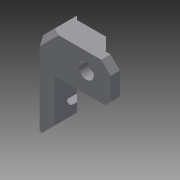
# Autodesk Inventor part: z-axis-top
Saved by Autodesk Inventor 2015 (Build 190159000, 159)
## iProperties
Created: 2015-05-31
Part Number: z-axis-top
Material: Generic
Document SubType Name: Modeling
Designer: X
Density: 1 g/cm^3
Appearance: Default
Author: X
Autodesk Inventor part; units mm, degrees
ref_plane "YZ Plane" through (0, 0, 0) normal (1, 0, 0) x (0, 1, 0)
ref_plane "XZ Plane" through (0, 0, 0) normal (0, 1, 0) x (-1, 0, 0)
ref_plane "XY Plane" through (0, 0, 0) normal (0, 0, 1) x (1, 0, 0)
sketch "Sketch1" plane through (0, 0, 0) normal (0, 1, 0) x (-1, 0, 0)
  line L0 (0, 0) -> (38, 0)
  line L1 (38, 0) -> (38, -50)
  line L2 (38, -50) -> (0, -50)
  line L3 (0, -50) -> (0, 0)
  dimension "d0" = 38
  dimension "d1" = 50
  constraints: 8 end point, 2 parallel, 1 horizontal, 1 perpendicular
  measures "d0" distance of L0.start L0.end
  measures "d1" distance of L2.end L0.start
extrude "Extrusion1" add sketch "Sketch1" along normal blind 16
sketch "Sketch2" plane through (0, 16, 0) normal (0, 1, 0) x (1, 0, 0)
  line L0 (0, 50) -> (-30, 50)
  line L1 (-30, 50) -> (-30, 20)
  line L2 (-30, 20) -> (0, 20)
  line L3 (0, 20) -> (0, 50)
  line L4 (-38, 50) -> (-38, 0) projected
  line L5 (0, 0) -> (-38, 0) projected
  dimension "d4" = 8
  dimension "d5" = 20
  constraints: 8 end point, 2 parallel, 1 horizontal, 1 perpendicular
  measures "d4" distance between parallel lines of L1 L4
  measures "d5" distance between parallel lines of L5 L2
extrude "Extrusion2" cut sketch "Sketch2" against normal through all
sketch "Sketch3" plane through (0, 16, 0) normal (0, 1, 0) x (1, 0, 0)
  line L0 (0, 20) -> (-30, 20)
  line L1 (-30, 20) -> (-30, 5)
  line L2 (-30, 5) -> (0, 5)
  line L3 (0, 5) -> (0, 20)
  line L4 (-30, 20) -> (-30, 50) projected
  line L5 (-38, 0) -> (0, 0) projected
  dimension "d8" = 5
  constraints: 8 end point, 2 parallel, 1 collinear, 1 horizontal, 1 perpendicular
  measures "d8" distance between parallel lines of L5 L2
extrude "Extrusion3" cut sketch "Sketch3" against normal blind 11
sketch "Sketch4" plane through (-38, 0, 0) normal (0, 0, 1) x (1, 0, 0)
  line L0 (4, 16) -> (8, 12)
  line L1 (8, 12) -> (23.5, 12)
  line L2 (23.5, 12) -> (30, 5.5)
  line L3 (30, 5.5) -> (30, 5)
  line L4 (30, 5) -> (38, 5)
  line L5 (4, 16) -> (38, 16)
  line L6 (38, 5) -> (38, 16) projected
  line L7 (38, 16) -> (38, 5)
  line L8 (0, 16) -> (38, 16) projected
  line L9 (38, 0) -> (38, 16) projected
  line L10 (38, 0) -> (0, 0) projected
  line L11 (0, 0) -> (0, 16) projected
  dimension "d11" = 0.5
  dimension "d12" = 8
  dimension "d13" = 5
  dimension "d16" = 7
  dimension "d17" = 15.5
  dimension "d18" = 8
  dimension "d19" = 4
  constraints: 14 end point, 2 perpendicular, 1 collinear, 1 horizontal, 1 parallel, 1 point on line, 1 vertical
  measures "d11" distance of L2.end L3.end
  measures "d12" distance of L3.end L4.end
  measures "d13" distance between parallel lines of L10 L4
  measures "d16" distance from line of L3.end L1
  measures "d17" distance of L0.end L1.end
  measures "d18" distance from line of L11 L0.end
  measures "d19" distance from line of L11 L0.start
extrude "Extrusion4" cut sketch "Sketch4" against normal through all contours L5 L6 L4 L3 L2 L1 L0
chamfer "Chamfer1" distance 7 distance2 7 1 edges at (-30, 6, -50) measured on face at (-30.5, 6, -50)
chamfer "Chamfer2" distance 6 distance2 6 1 edges at (-38, 8, 0) measured on face at (-38, 8, -0.5)
chamfer "Chamfer3" distance 1 distance2 1 1 edges at (-38, 8, -50) measured on face at (-37.5, 8, -50)
chamfer "Chamfer4" distance 5 distance2 5 1 edges at (0, 2.5, 0) measured on face at (-0.5, 2.5, 0)
chamfer "Chamfer5" distance 3 distance2 3 1 edges at (0, 2.5, -20) measured on face at (0, 2.5, -19.5)
chamfer "Chamfer6" distance 2 distance2 3 1 edges at (-35, 0, -3) measured on face at (-35, 0.5, -3)
sketch "Sketch5" plane through (-30, 0, -20) normal (1, 0, 0) x (0, 0, -1)
  line L0 (-5, 10) -> (15, 10) construction
  line L1 (-18, 16) -> (27, 16) construction
  line L2 (-20, 5.5) -> (-20, 12) construction
  line L3 (-15, 12) -> (-15, 5) projected
  point P0 (-20, 0)
  dimension "d40" = 6
  dimension "d41" = 20
  dimension "d45" = 10
  constraints: 2 end point, 1 horizontal, 1 parallel
  measures "d40" distance between parallel lines of L0 L1
  measures "d41" distance of L0.end L0.start
  measures "d45" distance from line of L3 L0.start
hole "Hole1" at (-30, 10, -15) at (-30, 10, -35) direction (-1, 0, 0) diameter 3.6 end through all counterbore diameter 6.2 counterbore depth 4
sketch "Sketch6" plane through (0, 16, 0) normal (0, 1, 0) x (1, 0, 0)
  line L0 (-30, 11.9) -> (-34, 11.9)
  line L1 (-34, 11.9) -> (-34, 18.1)
  line L2 (-34, 18.1) -> (-30, 18.1)
  line L3 (-30, 18.1) -> (-30, 11.9)
  line L4 (-30, 11.9) -> (-34, 18.1) construction
  line L5 (-34, 11.9) -> (-30, 18.1) construction
  line L6 (-30, 31.9) -> (-34, 31.9)
  line L7 (-34, 31.9) -> (-34, 38.1)
  line L8 (-34, 38.1) -> (-30, 38.1)
  line L9 (-30, 38.1) -> (-30, 31.9)
  line L10 (-30, 31.9) -> (-34, 38.1) construction
  line L11 (-34, 31.9) -> (-30, 38.1) construction
  line L12 (-32, 15) -> (-32, 35) construction
  line L13 (-38, 49) -> (-38, 6) construction
  line L14 (-30, 32.6315) -> (-30, 17.3685) construction
  point P0 (0, 0)
  point P1 (-30, 5)
  dimension "d53" = 6.2
  dimension "d54" = 6.2
  dimension "d55" = 20
  dimension "d56" = 4
  dimension "d57" = 10
  constraints: 26 end point, 5 parallel, 4 midpoint, 2 collinear, 2 horizontal, 2 perpendicular, 1 vertical
  measures "d53" distance between parallel lines of L2 L0
  measures "d54" distance of L6.end L7.end
  measures "d55" distance of L12.end L12.start
  measures "d56" distance of L0.start L0.end
  measures "d57" vertical distance of point (-30, 5) L12.start
extrude "Extrusion5" cut sketch "Sketch6" against normal blind 6
sketch "Sketch7" plane through (0, 5, 0) normal (0, 1, 0) x (1, 0, 0)
  line L0 (0, 17) -> (0, 5) projected
  line L1 (-30, 20) -> (-3, 20) projected
  point P0 (0, 0)
  point P1 (-13, 9.2)
  dimension "d60" = 13
  dimension "d61" = 10.8
  measures "d60" distance from line of L0 point (-13, 9.2)
  measures "d61" distance from line of L1 point (-13, 9.2)
hole "Hole2" at (-13, 5, -9.2) direction (0, -1, 0) diameter 8 end through all
equation "\"d53\" = d48"
equation "\"d54\" = d48"
equation "\"d55\" = d41"
equation "\"d57\" = d45"
equation "\"d48\" = 6.2"
body "Solid1"
